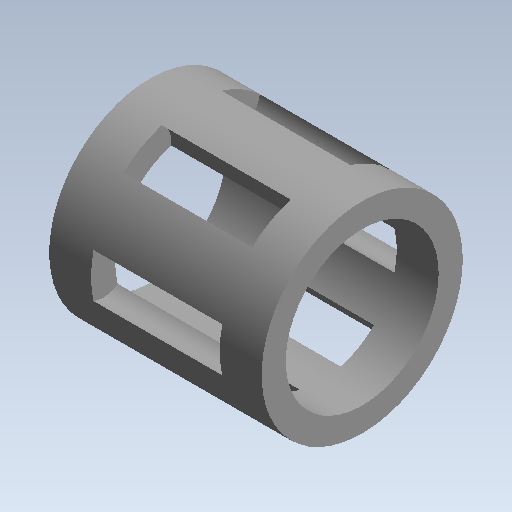
# Autodesk Inventor part: HK0408FT2CA
Saved by Autodesk Inventor 2021.3 (Build 253353010, 353A)
## iProperties
Category: PARTsolutions
Company: NTN
Part Number: HK0408FT2CA
Material: 一般
Catalog Web Link: www.cadenas.de
Description: Needle Roller Shell Bearings open-ended CA-
Vendor: NTN
Document SubType Name: Modeling
Designer: partserver
Manufacturer: NTN
Mass: 0.0596463 g
Surface Area: 2.42578 cm^2
Volume: 0.0596463 cm^3
Density: 1 g/cm^3
Appearance: PSOLRGB-192-192-192
PSOL_IDENT_0: {$CADENAS_DATA\23d-libs\ntn\needle_roler_bearings\needle_roller_shell_bearings_open_ended_ca.prj},19
PSOL_IDENT_1: 8 {VTYP=3D},{NB=HK0408FT2CA},{LINA=HK0408FT2CA},{NN=Needle Roller Shell Bearings open-ended CA},{DAT
PSOL_IDENT_2: E=23.10.2020 01:12:35},{GEOMDATE=20.04.2020 08:33:10},{VERSION=},{LINEID=20},{WBVAR=},{WBNUMERIC=}
PSOL_IDENT_3: {NB=HK0408FT2CA},{LINA=HK0408FT2CA},{KT=DUMMY},{FW=4},{D=8.0},{C=8},{ORDER=HK0408FT2},{CR=1770},{COR=
PSOL_IDENT_4: 1270},{CRF=180},{CORF=129},{LSG=30000},{LSO=45000},{MASS=0.0016},{IT=-},{RT=1.6},{VER=1},{T=0.500},{
PSOL_IDENT_5: DW=1.500},{LW=4.000},{NR=6.000},{CID=4.750},{CD=6.250},{CW=6.600},{SD=4.200}
NB: HK0408FT2CA
NN: Needle Roller Shell Bearings open-ended CA
NBSYN: $ORDER.CA
LINA: HK0408FT2CA
CATALOG: NTN Corporation
FW: 4
D: 8
C: 8
ORDER: HK0408FT2
CR: 1770
COR: 1270
CRF: 180
CORF: 129
LSG: 30000
LSO: 45000
MASS: 0.0016
IT: -
RT: 1.6
VER: 1
SUPPLIER: NTN
ARTICLENO: HK0408FT2CA
BOMINFO: HK0408FT2CA
CREATOR: CADENAS GmbH
Title: HK0408FT2CA
Author: Cadenas PARTsolutions
Autodesk Inventor part; units mm, degrees
sketch "Sketch_1" plane through (0, 0, 0) normal (0, 0, 1) x (1, 0, 0)
  line L0 (7.3, 0) -> (0.7, 0)
  line L1 (0.7, 2.375) -> (7.3, 2.375)
  line L2 (7.3, 2.375) -> (7.3, 3.125)
  line L3 (7.3, 3.125) -> (0.7, 3.125)
  line L4 (0.7, 3.125) -> (0.7, 2.375)
  constraints: 10 end point
revolve "Revolution1" add sketch "Sketch_1" angle 360 about axis through (7.3, 0, 0) along (1, 0, 0)
sketch "Sketch_2" plane through (0, 0, 0) normal (0, 0, 1) x (1, 0, 0)
  line L0 (6, 2.75) -> (2, 2.75)
  line L1 (2, 2.75) -> (2, 3.5)
  line L2 (2, 3.5) -> (6, 3.5)
  line L3 (6, 3.5) -> (6, 2.75)
  line L4 (6, 2.75) -> (2, 2.75)
  constraints: 10 end point
revolve "Revolution2" cut sketch "Sketch_2" angle 360 about axis through (6, 2.75, 0) along (1, 0, 0)
pattern_linear "Rectangular Pattern1" count 3 spacing 2.75 along (0, -0.5, 0.866) count 3 spacing 2.75 along (0, -0.5, -0.866) of "Revolution2"
ref_plane "IP_1_XY" through (4, 0, 0) normal (1, 0, 0) x (0, 0, -1)
ref_plane "IP_1_YZ" through (4, 0, 0) normal (0, 0, -1) x (0, 1, 0)
ref_plane "IP_1_ZX" through (4, 0, 0) normal (0, 1, 0) x (1, 0, 0)
ref_plane "IP_3_1_XY" through (4, 2.75, 0) normal (1, 0, 0) x (0, 0, -1)
ref_plane "IP_3_1_YZ" through (4, 2.75, 0) normal (0, 0, -1) x (0, 1, 0)
ref_plane "IP_3_1_ZX" through (4, 2.75, 0) normal (0, 1, 0) x (1, 0, 0)
ref_plane "IP_3_2_XY" through (4, 1.375, 2.3816) normal (1, 0, 0) x (0, 0, -1)
ref_plane "IP_3_2_YZ" through (4, 1.375, 2.3816) normal (0, 0, -1) x (0, 1, 0)
ref_plane "IP_3_2_ZX" through (4, 1.375, 2.3816) normal (0, 1, 0) x (1, 0, 0)
ref_plane "IP_3_3_XY" through (4, -1.375, 2.3816) normal (1, 0, 0) x (0, 0, -1)
ref_plane "IP_3_3_YZ" through (4, -1.375, 2.3816) normal (0, 0, -1) x (0, 1, 0)
ref_plane "IP_3_3_ZX" through (4, -1.375, 2.3816) normal (0, 1, 0) x (1, 0, 0)
ref_plane "IP_3_4_XY" through (4, -2.75, 0) normal (1, 0, 0) x (0, 0, -1)
ref_plane "IP_3_4_YZ" through (4, -2.75, 0) normal (0, 0, -1) x (0, 1, 0)
ref_plane "IP_3_4_ZX" through (4, -2.75, 0) normal (0, 1, 0) x (1, 0, 0)
ref_plane "IP_3_5_XY" through (4, -1.375, -2.3816) normal (1, 0, 0) x (0, 0, -1)
ref_plane "IP_3_5_YZ" through (4, -1.375, -2.3816) normal (0, 0, -1) x (0, 1, 0)
ref_plane "IP_3_5_ZX" through (4, -1.375, -2.3816) normal (0, 1, 0) x (1, 0, 0)
ref_plane "IP_3_6_XY" through (4, 1.375, -2.3816) normal (1, 0, 0) x (0, 0, -1)
ref_plane "IP_3_6_YZ" through (4, 1.375, -2.3816) normal (0, 0, -1) x (0, 1, 0)
ref_plane "IP_3_6_ZX" through (4, 1.375, -2.3816) normal (0, 1, 0) x (1, 0, 0)
body "Solid1"
